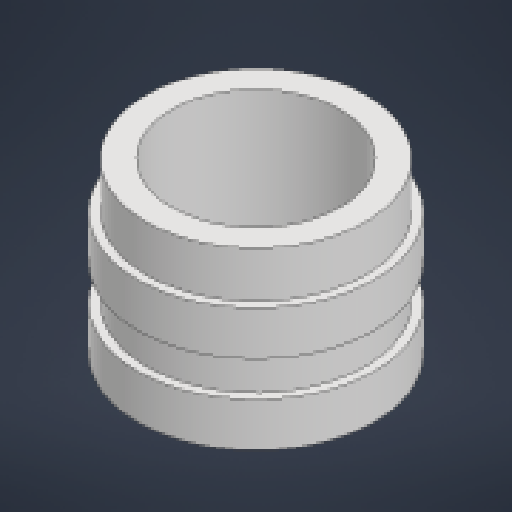
# Autodesk Inventor part: M5 heat set inserts
Saved by Autodesk Inventor 2026.1 (Build 301233020, 233B)
## iProperties
Created: 2025-09-22
Part Number: M5 heat set inserts
Material: Generic
Document SubType Name: Modeling
Designer: gavin
Density: 1 g/cm^3
Appearance: Default
Author: gavin
Autodesk Inventor part; units mm, degrees
ref_plane "YZ Plane" through (0, 0, 0) normal (1, 0, 0) x (0, 1, 0)
ref_plane "XZ Plane" through (0, 0, 0) normal (0, 1, 0) x (-1, 0, 0)
ref_plane "XY Plane" through (0, 0, 0) normal (0, 0, 1) x (1, 0, 0)
sketch "Sketch1" plane through (0, 0, 0) normal (1, 0, 0) x (0, 1, 0)
  line L0 (0, 0) -> (0, -3.5)
  line L1 (0, -3.5) -> (1.3, -3.5)
  line L2 (1.3, -3.5) -> (1.3, -3.25)
  line L3 (1.3, -3.25) -> (2.3425, -3.25)
  line L4 (2.3425, -3.25) -> (2.3425, -3.5)
  line L5 (2.3425, -3.5) -> (3.6425, -3.5)
  line L6 (3.6425, -3.5) -> (3.6425, -3.25)
  line L7 (3.6425, -3.25) -> (5, -3.25)
  line L8 (5, -3.25) -> (5, 0)
  line L9 (5, 0) -> (0, 0)
  line L10 (5, -2.5) -> (0, -2.5)
  point P0 (1.8212, -3.25)
  dimension "d0" = 3.25
  dimension "d1" = 5
  dimension "d2" = 3.5
  dimension "d3" = 1.3
  dimension "d4" = 1.3
  dimension "d5" = 2.5
  constraints: 22 end point, 6 perpendicular, 4 point on line, 2 horizontal, 2 parallel, 1 midpoint, 1 vertical
  measures "d0" distance between parallel lines of L9 L7
  measures "d1" distance of L8.end L0.start
  measures "d2" distance between parallel lines of L9 L1
  measures "d3" distance of L0.end L1.end
  measures "d4" distance of L4.end L5.end
  measures "d5" distance between parallel lines of L9 L10
revolve "Revolution1" add sketch "Sketch1" angle 360 about axis through (0, 5, 0) along (0, -1, 0) contours L10 L8 L7 L6 L5 L4 L3 L2 L1 L0
equation "\"d4\" = d3"
body "Solid1"
